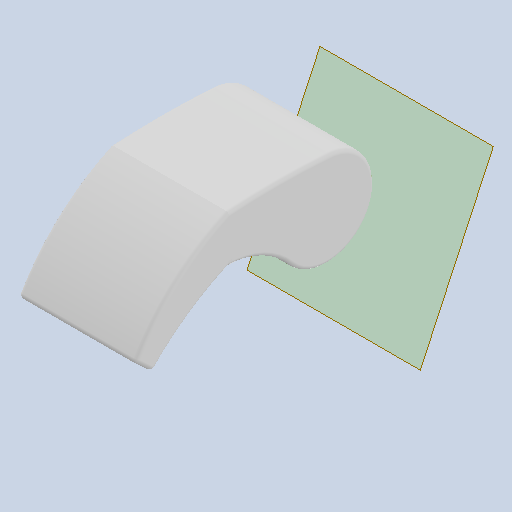
# Autodesk Inventor part: Hand
Saved by Autodesk Inventor 2025.2 (Build 292293000, 293)
## iProperties
Created: 2025-02-22
Part Number: Hand
Material: Generic
Document SubType Name: Modeling
Designer: andre
Density: 1 g/cm^3
Appearance: Default
Author: andre
Autodesk Inventor part; units mm, degrees
ref_plane "YZ Plane" through (0, 0, 0) normal (1, 0, 0) x (0, 1, 0)
ref_plane "XZ Plane" through (0, 0, 0) normal (0, 1, 0) x (-1, 0, 0)
ref_plane "XY Plane" through (0, 0, 0) normal (0, 0, 1) x (1, 0, 0)
sketch "Sketch1" plane through (0, 0, 0) normal (1, 0, 0) x (0, 1, 0)
  circle A0 centre (0, 12.383218) radius 6
  arc A1 (6, 12.383218) -> (6, 24.882493) centre (-85.102152, 18.632855) ccw
  arc A2 (6, 24.882493) -> (-4.765359, 36.675515) centre (-17.550727, 14.194149) ccw
  line L0 (-4.765359, 36.675515) -> (-6.795305, 34.488152)
  arc A3 (0, 24.882493) -> (-6.795305, 34.488152) centre (-28.46576, 11.951458) ccw
  arc A4 (-3.873416, 16.965428) -> (0, 24.882493) centre (-10.89829, 25.308405) ccw
  point P0 (0, 0)
  dimension "d0" = 12
  constraints: 10 point on circle, 5 centre point, 2 end point
  measures "d0" diameter of A0
extrude "Extrusion1" add sketch "Sketch1" along normal blind 15
ref_plane "Work Plane1" through (15, -2.525817, 6.940769) normal (0, -0.4209695, -0.9070748) x (1, 0, 0)
sketch "Sketch2" plane through (15, -2.525817, 6.940769) normal (0, -0.4209695, -0.9070748) x (1, 0, 0)
  circle A0 centre (-7.5, 0.071427) radius 2.649
  line L0 (-15, -6) -> (-15, 6)
  line L1 (0, -6) -> (0, 6)
  point P0 (-15, -5.212957)
  point P1 (-15, 5.442449)
  point P2 (-15, -5.442449)
  point P3 (0, 5.442449)
  point P4 (0, -5.442449)
  dimension "d3" = 5.298
  dimension "d4" = 7.5
  dimension "d5" = 7.5
  constraints: 1 centre point
  measures "d3" diameter of A0
  measures "d4" distance from line of L0 A0.centre
  measures "d5" distance from line of L1 A0.centre
extrude "Extrusion2" cut sketch "Sketch2" against normal blind 8.25
fillet "Fillet1" radius 0.5 2 edges at (4.8511, -2.6068, 6.9791) (4.851, 0.8832, 14.456)
fillet "Fillet2" radius 0.5 14 edges at (0, -2.5258, 6.9408) (0, 6.2141, 18.6329) (0, -1.1014, 20.5153) (0, 1.5502, 31.6306) (0, -2.9417, 30.0079) (0, -5.7803, 35.5818) (15, 6.2141, 18.6329) (15, -2.5258, 6.9408) (15, -1.1014, 20.5153) (15, 1.5502, 31.6306) (15, -2.9417, 30.0079) (15, -5.7803, 35.5818) (7.5, -4.7654, 36.6755) (7.5, -6.7953, 34.4882)
equation "\"d4\" = d5"
body "Solid1"
